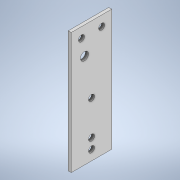
# Autodesk Inventor part: plateLocker
Saved by Autodesk Inventor 2020 (Build 240168000, 168)
## iProperties
Created: 2019-06-20
Part Number: plateLocker
Material: Generic
Document SubType Name: Modeling
Designer: Vivek Muskan
Density: 1 g/cm^3
Appearance: Default
Author: Vivek Muskan
Autodesk Inventor part; units mm, degrees
ref_plane "YZ Plane" through (0, 0, 0) normal (1, 0, 0) x (0, 1, 0)
ref_plane "XZ Plane" through (0, 0, 0) normal (0, 1, 0) x (-1, 0, 0)
ref_plane "XY Plane" through (0, 0, 0) normal (0, 0, 1) x (1, 0, 0)
sketch "Sketch1" plane through (0, 0, 0) normal (1, 0, 0) x (0, 1, 0)
  line L0 (0, 0) -> (-50, 0)
  line L1 (-50, 0) -> (-50, -20)
  line L2 (-50, -20) -> (0, -20)
  line L3 (0, -20) -> (0, 0)
  line L4 (0, 0) -> (0, -10)
  line L5 (0, -10) -> (-10, -10)
  line L6 (-10, -10) -> (-23, -10)
  line L7 (-23, -10) -> (-40, -10)
  line L8 (-40, -10) -> (-45, -10)
  circle A0 centre (-10, -10) radius 1.5
  circle A1 centre (-23, -10) radius 1.5
  circle A2 centre (-40, -10) radius 1.5
  circle A3 centre (-45, -10) radius 1.5
  dimension "d0" = 50
  dimension "d1" = 20
  dimension "d2" = 10
  dimension "d3" = 10
  dimension "d4" = 13
  dimension "d5" = 17
  dimension "d7" = 5
  dimension "d8" = 3
  dimension "d9" = 3
  dimension "d10" = 3
  dimension "d11" = 3
  constraints: 18 end point, 4 centre point, 4 coincident, 2 horizontal, 2 parallel, 2 perpendicular, 2 point on line, 1 midpoint
  measures "d0" distance of L2.end L1.end
  measures "d1" distance of L0.end L1.end
  measures "d2" distance of L0.start L4.end
  measures "d3" distance of L4.end L5.end
  measures "d4" distance of L5.end L6.end
  measures "d5" distance of L6.end L7.end
  measures "d7" distance of L7.end L8.end
  measures "d8" diameter of A0
  measures "d9" diameter of A1
  measures "d10" diameter of A2
  measures "d11" diameter of A3
extrude "Extrusion1" add sketch "Sketch1" along normal blind 1.5
sketch "Sketch2" plane through (0, 0, 0) normal (-1, 0, 0) x (0, 0, 1)
  line L0 (-20, 0) -> (0, 0) projected
  line L1 (0, 0) -> (-20, 0)
  line L2 (-20, 0) -> (-20, 10)
  line L3 (-20, 10) -> (0, 10)
  line L4 (0, 10) -> (0, 0)
  circle A0 centre (-10, -10) radius 1.5 projected
  line L5 (-10, -10) -> (-10, 5)
  line L6 (-10, 5) -> (-5, 5)
  line L7 (-5, 5) -> (-15, 5)
  circle A1 centre (-5, 5) radius 1.5
  circle A2 centre (-15, 5) radius 1.5
  dimension "d14" = 10
  dimension "d15" = 20
  dimension "d16" = 15
  dimension "d17" = 5
  dimension "d18" = 10
  dimension "d19" = 3
  dimension "d20" = 3
  constraints: 14 end point, 2 centre point, 2 coincident, 2 parallel, 2 perpendicular, 1 horizontal, 1 point on line, 1 vertical
  measures "d14" distance of L1.end L2.end
  measures "d15" distance of L2.end L3.end
  measures "d16" distance of L5.start L5.end
  measures "d17" distance of L5.end L6.end
  measures "d18" distance of L6.end L7.end
  measures "d19" diameter of A1
  measures "d20" diameter of A2
extrude "Extrusion2" add sketch "Sketch2" against normal blind 1.5 contours L2 L3 L4 L0
sketch "Sketch3" plane through (1.5, 0, 0) normal (1, 0, 0) x (0, 0, -1)
  circle A0 centre (10, -10) radius 1.5 projected
  circle A1 centre (10, -10) radius 1.5
  point P0 (0, 0)
  constraints: 1 centre point, 1 coincident
extrude "Extrusion3" add sketch "Sketch3" against normal blind 1.5
sketch "Sketch5" plane through (0, 0, 0) normal (-1, 0, 0) x (0, 0, 1)
  line L0 (0, 10) -> (0, -50) projected
  line L1 (0, 10) -> (0, -3.388)
  line L2 (0, -3.388) -> (-6.5, -3.388)
  circle A0 centre (-6.5, -3.388) radius 2
  point P0 (0, 0)
  dimension "d30" = 13.388
  dimension "d31" = 6.5
  dimension "d32" = 4
  constraints: 4 end point, 1 centre point, 1 coincident, 1 perpendicular, 1 point on line
  measures "d30" distance of L0.start L1.end
  measures "d31" distance of L1.end L2.end
  measures "d32" diameter of A0
extrude "Extrusion5" cut sketch "Sketch5" against normal blind 1.5
body "Solid1"
